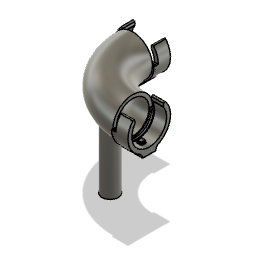
_Corner 7_5_2022.2632e461-b5ba-465b-90f7-7b59849efb52 (Autodesk Fusion 360 design; units mm, degrees)
Autodesk Fusion 360 part; units mm, degrees
note: some values were not read from the file. Set by a fixed rule: which face or edge a step refers to.
sketch "Sketch1" plane through (0, 0, 0) normal (0, 0, 1) x (1, 0, 0)
  circle A0 centre (0, 0) radius 16.875
  circle A1 centre (0, 0) radius 18.125
  circle A2 centre (0, 0) radius 15
  line L0 (33, 0) -> (-30, 0) construction
  line L1 (0, 29) -> (0, -23) construction
  arc A3 (-19.5, 0) -> (19.5, 0) centre (0, 0) ccw
  line L2 (15, 0) -> (19.5, 0)
  line L3 (-15, 0) -> (-19.5, 0)
  dimension "d8" = 33.75
  dimension "d9" = 1.25
  dimension "d50" = 30
  dimension "d95" = 19.5
  dimension "d96" = 4.5
  constraint coincident A0.centre A1.centre
  constraint horizontal L0
  constraint vertical L1
  constraint concentric A2 A3
  constraint coincident L0 A3.end
  constraint coincident L0 A3.start
  constraint coincident L0 L2.start
  constraint coincident A2 L2.start
  constraint coincident A2 L3.start
  constraint coincident L0 L3.start
  measures "d8" diameter of A0
  measures "d50" diameter of A2
  measures "d95" radius of A3
  measures "d96" distance of A3.end L2.start
sketch "Sketch2" plane through (0, 0, 0) normal (0, 1, 0) x (1, 0, 0)
  arc A0 (0, 0) -> (50, -50) centre (50, 0) ccw
  line L0 (50, 0) -> (0, 0) construction
  line L1 (50, 0) -> (50, -50) construction
  line L2 (50, 0) -> (14.6447, -35.3553)
  dimension "d1" = 90
  dimension "d10" = 50
  constraint coincident A0.start L0.end
  constraint coincident A0.centre L0.start
  constraint midpoint A0 L2.end
  measures "d1" angle of L0 L1
  measures "d10" radius of A0
sweep "Sweep2" add profiles "Sketch1" path "Sketch2" along A0 section 1 contours A0 A2 L2 L3 | A0 A1 L2 L3 | A0 A2 L2 L3 | A0 A1 L2 L3 makes body 1
ref_plane "WorkPlane5" through (0, 0, -4) normal (0, 0, -1) x (-1, 0, 0)
sketch "Sketch8" plane through (0, 0, -4) normal (0, 0, -1) x (1, 0, 0)
  line L0 (-6, 39.5) -> (-6, 21.8918)
  arc A0 (-8.7551, 17.4241) -> (-6, 21.8918) centre (-11, 21.8918) ccw
  arc A1 (13.1665, -9.3095) -> (13.3063, -11.9529) centre (22.1261, -10.161) ccw
  arc A2 (13.329, -8.8509) -> (13.1665, -9.3095) centre (14.162, -9.4041) ccw
  arc A3 (-15.0585, -12.3891) -> (-13.3063, -11.9529) centre (-14.2863, -11.7538) ccw
  line L1 (0, 39.5) -> (6, 39.5)
  arc A4 (-8.7551, 17.4241) -> (-15.0585, -12.3891) centre (0, 0) ccw
  arc A5 (-13.3063, -11.9529) -> (-13.1665, -9.3095) centre (-22.1261, -10.161) ccw
  line L2 (0, 0) -> (26.8441, -18.7964) construction
  line L3 (-8, 28.5277) -> (0, 28.5277)
  arc A6 (0, 16) -> (-13.329, -8.8509) centre (0, 0) ccw
  arc A7 (6, 21.8918) -> (8.7551, 17.4241) centre (11, 21.8918) ccw
  line L4 (6, 39.5) -> (6, 21.8918)
  line L5 (8, 28.5277) -> (0, 28.5277)
  line L6 (0, 50) -> (0, -42) construction
  arc A8 (13.329, -8.8509) -> (0, 16) centre (0, 0) ccw
  arc A9 (15.0585, -12.3891) -> (8.7551, 17.4241) centre (0, 0) ccw
  line L7 (28, 0) -> (20.2823, 0) construction
  line L8 (0, 39.5) -> (-6, 39.5)
  arc A10 (13.3063, -11.9529) -> (15.0585, -12.3891) centre (14.2863, -11.7538) ccw
  arc A11 (-13.1665, -9.3095) -> (-13.329, -8.8509) centre (-14.162, -9.4041) ccw
  line L9 (19.5, 0) -> (-24, 0) construction
  line L10 (11.1467, 16) -> (0, 16)
  line L11 (0, 16) -> (-11.1468, 16)
  line L12 (6, 21.8918) -> (-6, 21.8918)
  point P0 (0, 50)
  dimension "d54" = 32
  dimension "d55" = 6
  dimension "d56" = 39.5
  dimension "d57" = 3.5
  dimension "d58" = 5
  dimension "d59" = 55
  dimension "d60" = 1
  dimension "d61" = 9
  dimension "d62" = 1
  constraint coincident A4.centre L2.start
  constraint perpendicular L1 L4
  constraint coincident L1.start L6
  constraint coincident A6.start L6
  constraint tangent A7 A9
  constraint tangent A7 L4
  constraint coincident L3.end L6
  constraint perpendicular L5 L6
  constraint symmetric A4.centre L2.start L6
  constraint symmetric L1.start L8.start L6
  constraint symmetric L1.end L0.start L6
  constraint symmetric P0 L6.start L6
  constraint symmetric A6.start A8.end L6
  constraint symmetric A6 L6 A8
  constraint symmetric A4 L6 A9
  constraint symmetric L0.end A7.start L6
  constraint symmetric A0.start A7.end L6
  constraint symmetric A0 A7 L6
  constraint symmetric L3.start L5.start L6
  constraint symmetric L3.end L5.end L6
  constraint coincident L9.start A9
  constraint collinear L7 L9
  constraint tangent A9 A10
  constraint tangent A1 A10
  constraint tangent A1 A2
  constraint tangent A2 A8
  constraint equal A2 A10
  constraint symmetric A1 A5 L6
  constraint symmetric A3.start A9.start L6
  constraint symmetric A1.end A3.end L6
  constraint symmetric A3 L6 A10
  constraint tangent A5 A11
  constraint tangent A6 A11
  constraint coincident A9 L10.start
  constraint tangent A6 L10
  constraint coincident A4 L11.end
  constraint tangent A6 L11
  constraint perpendicular L6 L11
  constraint perpendicular L0 L12
  measures "d54" diameter of A8
  measures "d55" distance of L1.end L1.start
  measures "d56" distance of A4.centre L1
  measures "d57" distance of A8 A9
  measures "d58" radius of A7
  measures "d59" angle of L2 L6
  measures "d60" radius of A10
  measures "d61" radius of A1
  measures "d62" radius of A11
extrude "Extrude8" add sketch "Sketch8" against normal blind 8 separate body contours A0 A4 A7 A9 L10 L11 L12 makes body 2
extrude "Extrude9" add sketch "Sketch8" along normal blind 11.15 separate body contours A0 A4 A7 A9 L10 L11 L12 | A3 A4 A5 A6 A11 L11 | A1 A2 A8 A9 A10 L10 makes body 3
extrude "Extrude10" add sketch "Sketch1" against normal blind 3 separate body contours A0 A1 L2 L3 | A0 A2 L2 L3 | A1 A3 L2 L3 picked at (17.578, -1.7388) picked at (-13.8467, -8.4259) makes body 4
shell "Shell1" thickness 0.75 removed faces 7 at (-15.625, 0, -1) at (-17.2917, 0, -1) at (-18.5833, 0, -1) at (17.2917, 0, -1) at (15.625, 0, -1) at (18.5833, 0, -1) at (14.9814, -0.7477, -2) on bodies 4
ref_plane "WorkPlane6" through (0, -16, -4) normal (0, 1, 0) x (-1, 0, 0)
sketch "Sketch9" plane through (0, -16, -4) normal (0, 1, 0) x (1, 0, 0)
  line L0 (16, 0) -> (-16, 0)
  line L1 (13.329, 0) -> (13.329, 11.15)
  line L2 (-16, 11.15) -> (16, 11.15)
  line L3 (-13.329, 11.15) -> (-13.329, 0)
  line L4 (1.175, 1.754) -> (-1.175, 1.754)
  line L5 (-2.175, 2.754) -> (-2.175, 5.104)
  line L6 (-1.175, 6.104) -> (1.175, 6.104)
  line L7 (2.175, 5.104) -> (2.175, 2.754)
  arc A0 (1.175, 1.754) -> (2.175, 2.754) centre (1.175, 2.754) ccw
  arc A1 (-2.175, 2.754) -> (-1.175, 1.754) centre (-1.175, 2.754) ccw
  arc A2 (-1.175, 6.104) -> (-2.175, 5.104) centre (-1.175, 5.104) ccw
  arc A3 (2.175, 5.104) -> (1.175, 6.104) centre (1.175, 5.104) ccw
  point P0 (2.175, 1.754)
  point P1 (-2.175, 1.754)
  point P2 (2.175, 6.104)
  dimension "d71" = 4.35
  dimension "d72" = 4.35
  dimension "d73" = 1
  dimension "d74" = 2.175
  dimension "d75" = 1.754
  constraint horizontal L4
  constraint vertical L5
  constraint horizontal L6
  constraint vertical L7
  constraint coincident P0 L4
  constraint coincident P0 L7
  constraint tangent L4 A0
  constraint tangent L7 A0
  constraint coincident P1 L4
  constraint coincident P1 L5
  constraint tangent L4 A1
  constraint tangent L5 A1
  constraint equal A0 A1
  constraint tangent L6 A2
  constraint tangent L5 A2
  constraint equal A0 A2
  constraint coincident P2 L6
  constraint coincident P2 L7
  constraint tangent L6 A3
  constraint tangent L7 A3
  constraint equal A0 A3
  measures "d71" distance of P0 P1
  measures "d72" distance of P0 P2
  measures "d73" radius of A0
  measures "d74" distance of origin L5
  measures "d75" distance of L0 L4
extrude "Extrude11" add sketch "Sketch9" along normal blind 2 contours L4 L5 L6 L7 A0 A1 A2 A3 bodies 1 3 2 4
fillet "Fillet3" radius 0.4 9 faces at (-0.725, -14, -7.5373) (0, -14.6667, -10.104) (-1.2697, -14.6486, -10.0995) (-2.175, -15.2343, -7.5373) (-2.0375, -15.2458, -6.248) (0, -14.6667, -5.754) (1.2697, -14.6486, -5.7585) (2.175, -15.2343, -8.3207) (2.0376, -15.2458, -9.61) on bodies 3
combine "Combine2" operation add target body 3 tool bodies 4 2
copy_body "CopyPasteBodies1" bodies 3 makes body 5
copy_body "CopyPasteBodies2" bodies 3 makes body 6
copy_body "CopyPasteBodies3" bodies 3 makes body 7
copy_body "CopyPasteBodies4" bodies 3 makes body 8
move_body "Move1" bodies 8 to x (0, 0, 1) y (0, 1, 0) z (-1, 0, 0) at (-34.65, 0, 4.35)
move_body "Move2" bodies 8 to x (1, 0, 0) y (0, 1, 0) z (0, 0, 1) at (80.65, 0, 45.65)
move_body "Move3" bodies 8 to x (1, 0, 0) y (0, 1, 0) z (0, 0, 1) at (4, 0, 0)
ref_plane "WorkPlane8" through (0, -18.125, 0) normal (0, 1, 0) x (0, 0, 1)
sketch "Sketch13" plane through (0, -18.125, 0) normal (0, 1, 0) x (1, 0, 0)
  line L0 (50, 0) -> (14.6447, -35.3553)
  arc A0 (0, 0) -> (50, -50) centre (50, 0) ccw
  circle A1 centre (14.6447, -35.3553) radius 7.5
  dimension "d84" = 15
  constraint coincident L0.end A1.centre
  measures "d84" diameter of A1
extrude "Extrude13" add sketch "Sketch13" along normal up to surface and the other way blind 66.845 end surface at (37.1753, 3.5914, 66.541) on bodies 1 bodies 1
sketch "Sketch14" plane through (0, -84.97, 0) normal (0, -1, 0) x (1, 0, 0)
  circle A0 centre (14.6447, 35.3553) radius 7.5
  circle A1 centre (14.6447, 35.3553) radius 3.55
  line L0 (11.4259, 40.9303) -> (8.2072, 35.3553)
  line L1 (8.2072, 35.3553) -> (11.4259, 29.7803)
  line L2 (11.4259, 29.7803) -> (17.8634, 29.7803)
  line L3 (17.8634, 29.7803) -> (21.0821, 35.3553)
  line L4 (21.0821, 35.3553) -> (17.8634, 40.9303)
  line L5 (17.8634, 40.9303) -> (11.4259, 40.9303)
  point P0 (14.6447, 35.3553)
  point P1 (14.6447, 35.3553)
  dimension "d89" = 7.1
  dimension "d92" = 5.575
  constraint coincident P1 P0
  measures "d89" diameter of A1
  measures "d92" distance of P1 L5
extrude "Extrude14" cut sketch "Sketch14" against normal blind 35 contours A1 bodies 1
extrude "Extrude15" cut sketch "Sketch14" against normal blind 5.9 contours L0 L1 L2 L3 L4 L5 bodies 1
combine "Combine3" operation add target body 8 tool bodies 7 1
sketch "Sketch15" plane through (0, 0, -0.75) normal (0, 0, -1) x (-1, 0, 0)
  arc A0 (9.7756, -16) -> (18.75, 0) centre (0, 0) ccw
  line L0 (18.75, 0) -> (15, 0)
  arc A1 (-15, 0) -> (15, 0) centre (0, 0) ccw
  line L1 (-15, 0) -> (-18.75, 0)
  arc A2 (-18.75, 0) -> (-9.7756, -16) centre (0, 0) ccw
  circle A3 centre (0, 0) radius 18.5
  line L2 (0, -16) -> (9.7756, -16)
  line L3 (-9.7756, -16) -> (0, -16)
  dimension "d97" = 37
  constraint coincident A0.centre A1.centre
  measures "d97" diameter of A3
extrude "Extrude16" add sketch "Sketch15" along normal blind 1 separate body contours L0 A1 L1 A3 L2 L3 | A3 L2 L3 | L0 A1 L1 A3 makes body 9
ref_plane "WorkPlane9" through (0, 0, -1.25) normal (0, 0, 1) x (1, 0, 0)
sketch "Sketch16" plane through (0, 0, -1.25) normal (0, 0, 1) x (1, 0, 0)
  circle A0 centre (0, 0) radius 18.5
  line L0 (8, 16.6808) -> (8, 31.6808)
  line L1 (-8, 16.6808) -> (-8, 31.6808)
  line L2 (5.5, 36) -> (-5.5, 36)
  line L3 (-5.5, 36) -> (-5.5, 30)
  line L4 (-5.5, 30) -> (5.5, 30)
  line L5 (5.5, 30) -> (5.5, 36)
  line L6 (8, 31.6808) -> (8, 42)
  line L7 (8, 42) -> (-8, 42)
  line L8 (-8, 42) -> (-8, 31.6808)
  dimension "d100" = 15
  dimension "d101" = 15
  dimension "d102" = 8
  dimension "d103" = 8
  dimension "d104" = 11
  dimension "d105" = 6
  dimension "d106" = 6
  dimension "d107" = 42
  dimension "d108" = 2.5
  constraint coincident A0 L0.start
  constraint vertical L0
  constraint coincident A0 L1.start
  constraint parallel L0 L1
  constraint horizontal L2
  constraint vertical L3
  constraint horizontal L4
  constraint vertical L5
  constraint parallel L0 L6
  constraint perpendicular L1 L7
  constraint perpendicular L7 L8
  measures "d100" distance of L0.start L0.end
  measures "d101" distance of L1.start L1.end
  measures "d102" distance of A0.centre L0
  measures "d103" distance of A0.centre L1
  measures "d104" distance of L2.start L2.end
  measures "d105" distance of L2.start L4.end
  measures "d106" distance of L2 L7
  measures "d107" distance of A0.centre L7
  measures "d108" distance of L0 L5
extrude "Extrude17" add sketch "Sketch16" along normal up to surface (-0.5 mm away) and the other way up to surface (-0.5 mm away) contours A0 L0 L1 L6 L7 L8 bodies 9
move_face "MoveFace1" by (-93.6686, -60.9525, -102.5519) 2 faces at (2.7991, -3.3712, -0.75) (2.6739, 5.5693, -1.75) on bodies 9
extrude "Extrude18" add 1 faces at (53, -14.0163, 61.2444) along direction (1, 0, 0) blind 1 on bodies 8 bodies 8
extrude "Extrude19" add 1 faces at (11.2444, -14.0163, -3) along direction (0, 0, -1) blind 1 on bodies 8 bodies 8
hidden bodies 3 5 6 9
equation "d56 = 50 mm - 10.5 mm"
equation "d74 = d71 / 2"
equation "d87 = 74.845 mm - 8 mm"
equation "d92 = ( 11.25 / 2 ) * 1 mm - 0.05 mm"
equation "d103 = d102"
equation "d108 = ( d102 + d103 - d104 ) / 2"
